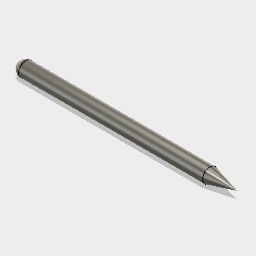
FPROJ_2 (Autodesk Fusion 360 design; units mm, degrees)
Autodesk Fusion 360 part; units mm, degrees
cylinder "圆柱体基本要素1" add diameter 8 height 100 placed x (0, 0, -1) y (0, 1, 0) z (1, 0, 0) at (0, 0, 0) makes body 1
sphere "球体基本要素1" add diameter 8 placed x (0, 0, -1) y (0, 1, 0) z (1, 0, 0) at (0, 30, 40) separate body makes body 2
move_body "对齐1" bodies 2 to x (0, 0, 1) y (0, 1, 0) z (-1, 0, 0) at (40, -30, 0)
sketch "草图5" plane through (0, 0, 0) normal (0, 1, 0) x (1, 0, 0)
  line L0 (-30, 15) -> (-34, 15)
  line L1 (-34, 15) -> (-34, 0)
  line L2 (-34, 0) -> (-30, 15)
revolve "旋转1" add sketch "草图5" angle 360 about axis through (-34, 0, -15) along (0, 0, 1) separate body makes body 3
move_face "MoveFace1" to x (0.866025, 0.5, 0) y (-0.5, 0.866025, 0) z (0, 0, 1) at (-4.5551, 17, 0) 1 faces at (-33.7889, 0.732, -15) on bodies 3
move_body "MoveFace2" bodies 3 to x (0.217854, 0.170331, -0.961003) y (0.584434, 0.765828, 0.268226) z (0.78165, -0.620077, 0.067292) at (-14.8682, -3.5099, -46.6647) on bodies 3
move_body "对齐2" bodies 3 to x (0.78165, 0, -0.623718) y (-0.620077, 0.107888, -0.777087) z (0.067292, 0.994163, 0.08433) at (127.5855, 14.9124, -19.9414)
combine "合并1" operation add target body 2 tool bodies 1 3
